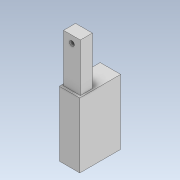
# Autodesk Inventor part: support_axe_radio
Saved by Autodesk Inventor 2020 (Build 240168000, 168)
## iProperties
Created: 2020-07-11
Part Number: support_axe_radio
Material: Generic
Document SubType Name: Modeling
Designer: Admin
Density: 1 g/cm^3
Appearance: Default
Author: Admin
Autodesk Inventor part; units mm, degrees
ref_plane "YZ Plane" through (0, 0, 0) normal (1, 0, 0) x (0, 1, 0)
ref_plane "XZ Plane" through (0, 0, 0) normal (0, 1, 0) x (-1, 0, 0)
ref_plane "XY Plane" through (0, 0, 0) normal (0, 0, 1) x (1, 0, 0)
sketch "Sketch1" plane through (0, 0, 0) normal (0, 1, 0) x (-1, 0, 0)
  line L0 (0, 0) -> (8.5, 0)
  line L1 (8.5, 0) -> (8.5, -17)
  line L2 (8.5, -17) -> (0, -17)
  line L3 (0, -17) -> (0, 0)
  dimension "d0" = 8.5
  dimension "d1" = 17
  constraints: 8 end point, 2 parallel, 1 horizontal, 1 perpendicular
  measures "d0" distance of L0.start L0.end
  measures "d1" distance of L2.end L0.start
extrude "Extrusion1" add sketch "Sketch1" along normal blind 27
sketch "Sketch2" plane through (0, 27, 0) normal (0, 1, 0) x (1, 0, 0)
  line L0 (-7.75, 1) -> (-0.75, 1)
  line L1 (-0.75, 1) -> (-0.75, 6)
  line L2 (-0.75, 6) -> (-7.75, 6)
  line L3 (-7.75, 6) -> (-7.75, 1)
  line L4 (-8.5, 0) -> (0, 0) projected
  line L5 (-8.5, 17) -> (-8.5, 0) projected
  dimension "d4" = 7
  dimension "d5" = 5
  dimension "d6" = 1
  dimension "d7" = 0.75
  constraints: 8 end point, 2 parallel, 1 horizontal, 1 perpendicular
  measures "d4" distance of L1.end L2.end
  measures "d5" distance of L2.end L0.start
  measures "d6" distance between parallel lines of L0 L4
  measures "d7" distance between parallel lines of L3 L5
extrude "Extrusion2" add sketch "Sketch2" along normal blind 20
sketch "Sketch3" plane through (-0.75, 27, -6) normal (0, 0, -1) x (-1, 0, 0)
  circle A0 centre (3.5, 17) radius 1
  line L0 (7, 0) -> (7, 20) projected
  line L1 (-0.75, 0) -> (7.75, 0) projected
  point P0 (-0.75, -27)
  dimension "d10" = 2
  dimension "d11" = 3.5
  dimension "d12" = 17
  constraints: 1 centre point
  measures "d10" diameter of A0
  measures "d11" distance from line of L0 A0.centre
  measures "d12" distance from line of L1 A0.centre
extrude "Extrusion3" cut sketch "Sketch3" against normal through all
body "Solid1"
